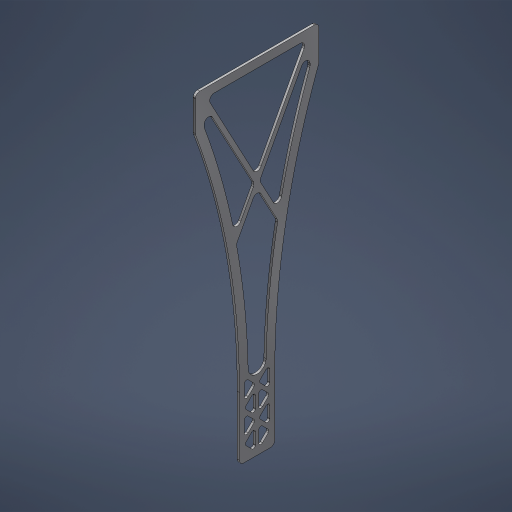
# Autodesk Inventor part: PLATE,ARM,TOP,TRIAL
Saved by Autodesk Inventor 2024.3 (Build 283343000, 343)
## iProperties
Category: _
Manager: _
ILogicPurgeVersion: 0.0.0.0
OnSaveVersion: 3.5.0.0
OnSaveAssembly: COREAutomationManager
Created: 2025-03-06
Part Number: PLATE,ARM,TOP,TRIAL
Checked By: 00
Engr Approved By: _
User Status: Work In Process
Material: Aluminum 3004-H32
Description: STANDARD (mm)
Document SubType Name: Sheet Metal
Mfg Approved By: John.Thibert
Designer: John.Thibert
Manufacturer: Standard
Standards Organization: Custom
Density: 2.71043 g/cm^3
Appearance: Aluminum - Polished
Sheet Metal Rule: Default
Mass: 161.594 g
Surface Area: 480.955 cm^2
Volume: 59.6194 cm^3
CN_MASS: 0.16
CN_SERVICEABLE: _
FIRST_DESCRIPTION: _
SECOND_DESCRIPTION: _
THIRD_DESCRIPTION: _
ModelCat: Uncategorized
MaterialName: Aluminum 3004-H32
Subject: _
Author: John.Thibert
Keywords: -
Revision Number: A
Autodesk Inventor part; units mm, degrees
ref_plane "YZ Plane" through (0, 0, 0) normal (1, 0, 0) x (0, 1, 0)
ref_plane "XZ Plane" through (0, 0, 0) normal (0, 1, 0) x (-1, 0, 0)
ref_plane "XY Plane" through (0, 0, 0) normal (0, 0, 1) x (1, 0, 0)
sketch "Sketch2" plane through (0, 0, 0) normal (1, 0, 0) x (0, 1, 0)
  line L0 (0, 88.9) -> (0, -88.9) construction
  line L1 (0, 88.9) -> (-25.4, 88.9)
  line L2 (0, 0) -> (-596.9, 0) construction
  line L3 (-378.953, 25.4) -> (-469.9, 25.4)
  line L4 (-469.9, 25.4) -> (-469.9, 0)
  line L5 (0, 88.9) -> (25.4, 88.9)
  line L6 (25.4, 88.9) -> (25.4, -88.9)
  line L7 (25.4, -88.9) -> (0, -88.9)
  line L8 (0, -88.9) -> (-25.4, -88.9)
  line L9 (-378.953, -25.4) -> (-469.9, -25.4)
  line L10 (-469.9, -25.4) -> (-469.9, 0)
  arc A0 (-378.953, 25.4) -> (-25.4, 88.9) centre (-378.953, 1041.4) ccw
  arc A1 (-25.4, -88.9) -> (-378.953, -25.4) centre (-378.953, -1041.4) ccw
  line L11 (-23.1263, 76.2) -> (12.7, 76.2)
  line L12 (12.7, 76.2) -> (12.7, -76.2)
  line L13 (12.7, -76.2) -> (-23.1263, -76.2)
  arc A2 (-23.1263, -76.2) -> (-355.8906, -12.9586) centre (-378.953, -1041.4) ccw
  arc A3 (-355.8906, 12.9586) -> (-23.1263, 76.2) centre (-378.953, 1041.4) ccw
  arc A4 (-355.8906, 12.9586) -> (-355.8906, -12.9586) centre (-355.6, 0) ccw
  point P0 (-155.3591, 37.2937)
  point P1 (12.7, -59.868)
  point P2 (-6.5384, -76.2)
  point P3 (-164.6377, 35.2725)
  dimension "d6" = 177.8
  dimension "d7" = 596.9
  dimension "d10" = 50.8
  dimension "d11" = 25.4
  dimension "d12" = 127
  dimension "d53" = 1016
  dimension "d54" = 12.7
  dimension "d65" = 355.6
  measures "d6" distance of L0.start L0.end
  measures "d7" distance of L2.start L2.end
  measures "d10" diameter of L3 L2
  measures "d11" distance of L6.end L0.end
  measures "d12" distance from line of L2.end L4
  measures "d53" radius of A0
  measures "d54" radial gap between concentric circles of A3 A0
  measures "d65" distance from line of A4.centre L0
extrude "Plate1" add sketch "Sketch2" along normal blind 3.175
sketch "Sketch5" plane through (3.175, 0, 0) normal (1, 0, 0) x (0, 0, -1)
  line L0 (-76.2, 12.7) -> (76.2, 12.7)
  line L1 (76.2, 12.7) -> (76.2, -23.1263)
  arc A0 (76.2, -23.1263) -> (12.9586, -355.8906) centre (1041.4, -378.953) ccw
  arc A1 (-12.9586, -355.8906) -> (12.9586, -355.8906) centre (0, -355.6) ccw
  arc A2 (-12.9586, -355.8906) -> (-76.2, -23.1263) centre (-1041.4, -378.953) ccw
  line L2 (-76.2, -23.1263) -> (-76.2, 12.7)
  line L3 (-88.9, -25.4) -> (-88.9, 25.4)
  arc A3 (-25.4, -378.953) -> (-88.9, -25.4) centre (-1041.4, -378.953) ccw
  line L4 (-25.4, -469.9) -> (-25.4, -378.953)
  line L5 (25.4, -469.9) -> (-25.4, -469.9)
  line L6 (25.4, -378.953) -> (25.4, -469.9)
  arc A4 (88.9, -25.4) -> (25.4, -378.953) centre (1041.4, -378.953) ccw
  line L7 (88.9, 25.4) -> (88.9, -25.4)
  line L8 (-88.9, 25.4) -> (88.9, 25.4)
  line L9 (76.2, 12.7) -> (-30.789, -186.8876) construction
  line L10 (-31.7412, -181.9436) -> (72.5976, 12.7)
  line L11 (76.2, 5.9797) -> (-29.8555, -191.8664)
  point P0 (0, 0)
  dimension "d59" = 6.35
  measures "d59" distance between parallel lines of L10 L11
sheet face with bend "Face2" sketch "Sketch5" thickness 3.175 toward (-1, 0, 0) bend radius 4.7625 contours L0 L1 L11 A2 L10
bend "Bend2"
mirror "Mirror2" about plane through (0, 0, 0) normal (0, 0, 1)
sketch "Sketch6" plane through (3.175, 0, 0) normal (1, 0, 0) x (0, 0, -1)
  line L0 (25.4, -469.9) -> (-25.4, -469.9) construction
  line L1 (0, -568.96) -> (0, 124.46) construction
  line L2 (-18.2563, -409.1898) -> (-18.2562, -440.9398)
  line L3 (-18.2562, -440.9398) -> (-2.3812, -425.0648)
  line L4 (-2.3812, -425.0648) -> (-18.2563, -409.1898)
  line L5 (-18.2562, -447.675) -> (-2.3812, -463.55)
  line L6 (-2.3812, -463.55) -> (-2.3812, -431.8)
  line L7 (-2.3812, -431.8) -> (-18.2562, -447.675)
  line L8 (-25.4, -469.9) -> (-25.4, -378.953) construction
  line L9 (-18.2563, -363.9694) -> (-18.2563, -395.7194)
  line L10 (-18.2563, -395.7194) -> (-2.3813, -379.8444)
  line L11 (-2.3813, -379.8444) -> (-18.2563, -363.9694)
  line L12 (-18.2563, -402.4546) -> (-2.3812, -418.3296)
  line L13 (-2.3812, -418.3296) -> (-2.3813, -386.5796)
  line L14 (-2.3813, -386.5796) -> (-18.2563, -402.4546)
  point P0 (0, 0)
  dimension "d67" = 15.875
  dimension "d68" = 2.3813
  dimension "d69" = 7.1437
  dimension "d70" = 4.7625
  dimension "d71" = 38.4852
  dimension "d72" = 6.7352
  dimension "d75" = 45.2204
  dimension "d80" = 6.35
  constraints: 24 end point, 4 point on line, 3 perpendicular, 2 parallel, 2 vertical, 12 other
  measures "d67" distance between parallel lines of L6 L2
  measures "d68" distance between parallel lines of L1 L6
  measures "d69" distance between parallel lines of L8 L2
  measures "d70" distance between parallel lines of L3 L7
  measures "d71" distance of L3.end L5.end
  measures "d72" distance of L3.end L6.end
  measures "d75" distance of L2.start L9.start
  measures "d80" distance from line of L5.end L0
extrude "Cut3" cut sketch "Sketch6" against normal blind 3.175
mirror "Mirror3" about plane through (0, 0, 0) normal (0, 0, 1) of "Cut3"
fillet "Corner Round3" radius 3.175 24 edges at (1.5875, -425.0648, 2.3812) (1.5875, -440.9398, 18.2562) (1.5875, -409.1898, 18.2563) (1.5875, -431.8, 2.3812) (1.5875, -463.55, 2.3812) (1.5875, -447.675, 18.2562) (1.5875, -386.5796, 2.3813) (1.5875, -418.3296, 2.3812) (1.5875, -402.4546, 18.2563) (1.5875, -379.8444, 2.3813) (1.5875, -395.7194, 18.2563) (1.5875, -363.9694, 18.2563) (1.5875, -440.9398, -18.2562) (1.5875, -425.0648, -2.3812) (1.5875, -409.1898, -18.2563) (1.5875, -463.55, -2.3812) (1.5875, -431.8, -2.3812) (1.5875, -447.675, -18.2562) (1.5875, -418.3296, -2.3812) (1.5875, -386.5796, -2.3813) (1.5875, -402.4546, -18.2563) (1.5875, -395.7194, -18.2563) (1.5875, -379.8444, -2.3813) (1.5875, -363.9694, -18.2563)
fillet "Corner Round2" radius 6.35 20 edges at (1.5875, -23.1263, -76.2) (1.5875, -23.1263, 76.2) (1.5875, 25.4, 88.9) (1.5875, -25.4, 88.9) (1.5875, 25.4, -88.9) (1.5875, -25.4, -88.9) (1.5875, -469.9, -25.4) (1.5875, -469.9, 25.4) (1.5875, 5.9797, 76.2) (1.5875, 12.7, 72.5976) (1.5875, -129.4508, 3.6024) (1.5875, -181.9436, 31.7412) (1.5875, -191.8664, 29.8555) (1.5875, -136.1711, 0) (1.5875, -191.8664, -29.8555) (1.5875, -181.9436, -31.7412) (1.5875, 5.9797, -76.2) (1.5875, 12.7, -72.5976) (1.5875, -129.4508, -3.6024) (1.5875, -122.7306, 0)
equation "\"d13\" = Thickness"
equation "\"BendRadius\" = 1.5 * Thickness"
equation "\"BendReliefWidth\" = Thickness"
equation "\"BendReliefDepth\" = 0.5 * Thickness"
equation "\"CornerReliefSize\" = 4 * Thickness"
equation "\"MinimumRemnant\" = 2 * Thickness"
equation "\"TransitionRadius\" = BendRadius"
equation "\"JacobiRadiusSize\" = BendRadius"
equation "\"GapSize\" = Thickness"
equation "\"Thickness\" = 3.175"
body "Solid2"
